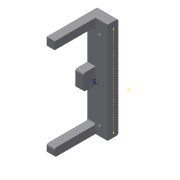
# Autodesk Inventor part: 30_Adapter_neje_to_cube_v3
Saved by Autodesk Inventor 2019.4 (Build 234330000, 330)
## iProperties
Created: 2021-04-09
Part Number: 30_Adapter_neje_to_cube_v3
Material: Generic
Document SubType Name: Modeling
Designer: UC2
Density: 1 g/cm^3
Appearance: Default
Author: UC2
Autodesk Inventor part; units mm, degrees
ref_plane "YZ Plane" through (0, 0, 0) normal (1, 0, 0) x (0, 1, 0)
ref_plane "XZ Plane" through (0, 0, 0) normal (0, 1, 0) x (-1, 0, 0)
sketch "Skizze1" plane through (0, 0, 0) normal (0, 0, 1) x (1, 0, 0)
  circle A0 centre (-23.32, -39.075) radius 2.355 construction
  circle A1 centre (-23.32, 39.075) radius 2.355 construction
  circle A2 centre (20.82, -6.975) radius 2 construction
  circle A3 centre (20.82, 7.075) radius 2 construction
  line L0 (32.82, 48.575) -> (-32.82, 48.575) construction
  arc A4 (-32.82, 48.575) -> (-34.82, 46.575) centre (-32.82, 46.575) ccw construction
  line L1 (-34.82, 46.575) -> (-34.82, -46.575) construction
  arc A5 (-34.82, -46.575) -> (-32.82, -48.575) centre (-32.82, -46.575) ccw construction
  line L2 (-32.82, -48.575) -> (32.82, -48.575) construction
  arc A6 (32.82, -48.575) -> (34.82, -46.575) centre (32.82, -46.575) ccw construction
  line L3 (34.82, -46.575) -> (34.82, 46.575) construction
  arc A7 (34.82, 46.575) -> (32.82, 48.575) centre (32.82, 46.575) ccw construction
  line L4 (-76.92, -46.575) -> (-35.32, -46.575) construction
  line L5 (-76.92, -40.695) -> (-76.92, -46.575) construction
  line L6 (-42.82, -40.695) -> (-76.92, -40.695) construction
  line L7 (-42.82, -0.875) -> (-42.82, -40.695) construction
  line L8 (-35.32, -0.875) -> (-42.82, -0.875) construction
  line L9 (-35.32, -46.575) -> (-35.32, -0.875) construction
  line L10 (-84.42, -46.575) -> (-76.92, -46.575) construction
  line L11 (-84.42, -0.875) -> (-84.42, -46.575) construction
  line L12 (-42.82, -0.875) -> (-84.42, -0.875) construction
  line L13 (-42.82, -6.755) -> (-42.82, -0.875) construction
  line L14 (-76.92, -6.755) -> (-42.82, -6.755) construction
  line L15 (-76.92, -46.575) -> (-76.92, -6.755) construction
  line L16 (-84.42, 3.425) -> (-76.92, 3.425) construction
  line L17 (-84.42, 49.125) -> (-84.42, 3.425) construction
  line L18 (-42.82, 49.125) -> (-84.42, 49.125) construction
  line L19 (-42.82, 43.245) -> (-42.82, 49.125) construction
  line L20 (-76.92, 43.245) -> (-42.82, 43.245) construction
  line L21 (-76.92, 3.425) -> (-76.92, 43.245) construction
  line L22 (-76.92, 3.425) -> (-35.32, 3.425) construction
  line L23 (-76.92, 9.305) -> (-76.92, 3.425) construction
  line L24 (-42.82, 9.305) -> (-76.92, 9.305) construction
  line L25 (-42.82, 49.125) -> (-42.82, 9.305) construction
  line L26 (-35.32, 49.125) -> (-42.82, 49.125) construction
  line L27 (-35.32, 3.425) -> (-35.32, 49.125) construction
  line L28 (-32.62, -40.5) -> (-32.62, -35.55) construction
  line L29 (-34.82, -40.5) -> (-32.62, -40.5) construction
  line L30 (-34.82, -35.55) -> (-32.62, -35.55) construction
  line L31 (-32.62, -11.9) -> (-32.62, -6.95) construction
  line L32 (-34.82, -11.9) -> (-32.62, -11.9) construction
  line L33 (-34.82, -6.95) -> (-32.62, -6.95) construction
  line L34 (-32.62, 9.5) -> (-32.62, 14.45) construction
  line L35 (-34.82, 9.5) -> (-32.62, 9.5) construction
  line L36 (-34.82, 14.45) -> (-32.62, 14.45) construction
  line L37 (-32.62, 38.1) -> (-32.62, 43.05) construction
  line L38 (-34.82, 38.1) -> (-32.62, 38.1) construction
  line L39 (-34.82, 43.05) -> (-32.62, 43.05) construction
  circle A8 centre (20.82, 7.075) radius 2 construction
  circle A9 centre (20.82, -6.975) radius 2 construction
  line L40 (13.32, -15) -> (17.82, -15) construction
  line L41 (13.32, -9.975) -> (13.32, -15) construction
  line L42 (17.32, -9.975) -> (13.32, -9.975) construction
  line L43 (17.32, -3.975) -> (17.32, -9.975) construction
  line L44 (13.32, -3.975) -> (17.32, -3.975) construction
  line L45 (13.32, 4.075) -> (13.32, -3.975) construction
  line L46 (17.32, 4.075) -> (13.32, 4.075) construction
  line L47 (17.32, 10.075) -> (17.32, 4.075) construction
  line L48 (13.32, 10.075) -> (17.32, 10.075) construction
  line L49 (13.32, 15) -> (13.32, 10.075) construction
  line L50 (17.82, 15) -> (13.32, 15) construction
  line L51 (17.82, 11) -> (17.82, 15) construction
  line L52 (23.82, 11) -> (17.82, 11) construction
  line L53 (23.82, 15) -> (23.82, 11) construction
  line L54 (28.32, 15) -> (23.82, 15) construction
  line L55 (28.32, 10.075) -> (28.32, 15) construction
  line L56 (24.32, 10.075) -> (28.32, 10.075) construction
  line L57 (24.32, 4.075) -> (24.32, 10.075) construction
  line L58 (28.32, 4.075) -> (24.32, 4.075) construction
  line L59 (28.32, -3.975) -> (28.32, 4.075) construction
  line L60 (24.32, -3.975) -> (28.32, -3.975) construction
  line L61 (24.32, -9.975) -> (24.32, -3.975) construction
  line L62 (28.32, -9.975) -> (24.32, -9.975) construction
  line L63 (28.32, -15) -> (28.32, -9.975) construction
  line L64 (23.82, -15) -> (28.32, -15) construction
  line L65 (23.82, -11) -> (23.82, -15) construction
  line L66 (17.82, -11) -> (23.82, -11) construction
  line L67 (17.82, -15) -> (17.82, -11) construction
  line L68 (-19.82, 48.575) -> (-34.82, 48.575)
  line L69 (-34.82, 48.575) -> (-34.82, -48.575)
  line L70 (-34.82, -48.575) -> (-19.82, -48.575)
  line L71 (-14.82, -43.575) -> (-14.82, 43.575)
  circle A10 centre (-23.32, 39.075) radius 2.455
  circle A11 centre (-23.32, -39.075) radius 2.255
  arc A12 (-19.82, -48.575) -> (-14.82, -43.575) centre (-19.82, -43.575) ccw
  arc A13 (-14.82, 43.575) -> (-19.82, 48.575) centre (-19.82, 43.575) ccw
  point P0 (0, 0)
  point P1 (-14.82, 48.575)
  point P2 (-14.82, -48.575)
  dimension "d1" = 0.1
  dimension "d2" = 0.1
  dimension "d8" = 20
  dimension "d9" = 5
  constraints: 24 end point, 9 horizontal, 5 point on line, 4 centre point, 4 point on circle, 4 tangent, 2 parallel, 1 collinear, 1 equal radius, 1 perpendicular, 1 vertical, 9 other
  measures "d1" radial gap between concentric circles of A1 A10
  measures "d2" radial gap between concentric circles of A0 A11
  measures "d8" distance between parallel lines of L71 L69
  measures "d9" radius of A12
extrude "Extrusion1" add sketch "Skizze1" along normal blind 5
sketch "Skizze2" plane through (0, 0, 5) normal (0, 0, 1) x (1, 0, 0)
  circle A0 centre (-23.32, 39.075) radius 2.455 construction
  circle A1 centre (-23.32, -39.075) radius 2.255 construction
  line L0 (-19.82, 48.575) -> (-34.82, 48.575) construction
  line L1 (-34.82, 48.575) -> (-34.82, -48.575) construction
  line L2 (-34.82, -48.575) -> (-19.82, -48.575) construction
  line L3 (-14.82, -43.575) -> (-14.82, 43.575) construction
  line L4 (-34.82, 48.575) -> (-29.82, 48.575)
  line L5 (-29.82, 48.575) -> (-29.82, -48.575)
  line L6 (-29.82, -48.575) -> (-34.82, -48.575)
  line L7 (-34.82, -48.575) -> (-34.82, 48.575)
  arc A2 (-19.82, -48.575) -> (-14.82, -43.575) centre (-19.82, -43.575) ccw projected
  arc A3 (-14.82, 43.575) -> (-19.82, 48.575) centre (-19.82, 43.575) ccw projected
  point P0 (0, 0)
  dimension "d5" = 5
  constraints: 8 end point, 2 parallel, 1 horizontal, 1 perpendicular, 1 point on line
  measures "d5" distance between parallel lines of L1 L5
ref_plane "Arbeitsebene1" through (-76.92, -46.575, 102.485) normal (0, 0, 1) x (1, 0, 0)
sketch "Sketch4" plane through (-34.82, -48.575, 0) normal (-1, 0, 0) x (0, 0, 1)
  line L0 (0, 0) -> (0, 97.15) projected
  line L1 (0, 0) -> (5, 0) projected
  line L2 (5, 97.15) -> (5, 0) construction
  line L3 (0, 97.15) -> (5, 97.15) projected
  circle A0 centre (41.935, 4.19) radius 2.475 projected
  circle A1 centre (13.335, 4.19) radius 2.475 projected
  circle A2 centre (13.335, 45.51) radius 2.475 projected
  circle A3 centre (13.335, 54.19) radius 2.475 projected
  circle A4 centre (13.335, 95.51) radius 2.475 projected
  circle A5 centre (41.935, 95.51) radius 2.475 projected
  line L4 (5, 0) -> (51, 0)
  line L5 (51, 0) -> (51, 8)
  line L6 (51, 8) -> (5, 8)
  line L7 (5, 8) -> (5, 0)
  line L8 (5, 8) -> (10.665, 8)
  line L9 (10.665, 8) -> (10.665, 99.5)
  line L10 (10.665, 99.5) -> (5, 99.5)
  line L11 (10.665, 99.5) -> (51, 99.5)
  line L12 (51, 99.5) -> (51, 91.82)
  line L13 (51, 91.82) -> (10.665, 91.82)
  line L14 (10.665, 91.82) -> (10.665, 99.5)
  line L15 (10.665, 41.82) -> (44.605, 41.82) projected
  line L16 (44.605, 57.88) -> (10.665, 57.88) projected
  line L17 (10.665, 41.82) -> (22.665, 41.82)
  line L18 (22.665, 41.82) -> (22.665, 57.88)
  line L19 (22.665, 57.88) -> (10.665, 57.88)
  line L20 (10.665, 57.88) -> (10.665, 41.82)
  line L21 (0, 0) -> (0, 97.15) projected
  line L22 (5, 99.5) -> (0, 99.5)
  line L23 (0, 99.5) -> (0, 0)
  line L24 (0, 0) -> (5, 0)
  line L25 (10.665, 91.82) -> (10.665, 57.88) construction
  line L26 (44.605, 91.82) -> (10.665, 91.82) construction
  line L27 (4.785, 99.7) -> (50.485, 99.7) construction
  line L28 (44.605, 91.82) -> (10.665, 91.82) construction
  circle A6 centre (6.975, 10.55) radius 2.475 projected
  circle A7 centre (6.975, 39.15) radius 2.475 projected
  circle A8 centre (6.975, 60.55) radius 2.475 projected
  circle A9 centre (6.975, 89.15) radius 2.475 projected
  line L29 (5, 97.15) -> (5, 0) projected
  line L30 (5, 40.6416) -> (5, 59.0584)
  line L31 (5, 59.0584) -> (5, 40.6416)
  line L32 (5, 62.0416) -> (5, 87.6584)
  line L33 (5, 90.6416) -> (5, 99.5)
  line L34 (5, 99.5) -> (5, 90.6416)
  line L35 (5, 87.6584) -> (5, 62.0416)
  line L36 (5, 37.6584) -> (5, 12.0416)
  line L37 (5, 9.0584) -> (5, 8)
  line L38 (5, 0) -> (5, 9.0584)
  line L39 (5, 12.0416) -> (5, 37.6584)
  point P0 (0, 48.575)
  dimension "d10" = 46
  dimension "d11" = 8
  dimension "d13" = 91.5
  dimension "d15" = 12
  constraints: 56 end point, 18 parallel, 8 point on circle, 5 horizontal, 5 perpendicular, 4 point on line, 2 coincident, 3 other
  measures "d10" distance of L6.end L5.end
  measures "d11" distance of L5.end L4.end
  measures "d13" distance of L9.end L8.end
  measures "d15" distance of L19.end L18.end
extrude "Extrusion3" add sketch "Sketch4" against normal up to surface (20 mm away) contours L0 L3 L29 A9 A8 A7 A6 L7 L1 | L23 L22 L33 L3 | L7 L6 L5 L4 | L33 L10 L9 L6 L29 A6 A7 A8 A9 | L29 A9 | L11 L12 L13 L9 | L9 L16 L18 L15 picked at (4.8333, 89.15)
fillet "Fillet1" radius 2 8 edges at (-24.82, 43.245, 10.665) (-24.82, 9.305, 22.665) (-24.82, -6.755, 22.665) (-24.82, -40.575, 10.665) (-24.82, -40.575, 51) (-24.82, -48.575, 51) (-24.82, 50.925, 0) (-24.82, -48.575, 0)
sketch "Sketch6" plane through (-34.82, -48.575, 2) normal (0, -1, 0) x (1, 0, 0)
  line L0 (20, 0) -> (0, 0) projected
  line L1 (20, 0) -> (20, 47) projected
  line L2 (0, 47) -> (20, 47) projected
  line L3 (0, 0) -> (0, 47) projected
  line L4 (20, 8.665) -> (0, 8.665) projected
  line L5 (0, 8.665) -> (20, 8.665) projected
  line L6 (21.8604, 55.0402) -> (8, 55.0402)
  line L7 (8, 55.0402) -> (8, 8.665)
  line L8 (8, 8.665) -> (21.8604, 8.665)
  line L9 (21.8604, 8.665) -> (21.8604, 55.0402)
  point P0 (34.82, -2)
  point P1 (12.8077, 8.665)
  dimension "d23" = 8
  constraints: 8 end point, 2 parallel, 1 horizontal, 1 perpendicular, 1 point on line
  measures "d23" distance between parallel lines of L7 L3
extrude "Extrusion5" cut sketch "Sketch6" against normal through all contours L4 L7 L2 L1 | L1 L2 L7 L6 L9 L8
sketch "Sketch7" plane through (-34.82, 43.245, 51) normal (-1, 0, 0) x (0, 0, 1)
  circle A0 centre (-37.665, -87.63) radius 2.475 projected
  circle A1 centre (-9.065, -87.63) radius 2.475 projected
  circle A2 centre (-37.665, -46.31) radius 2.475 projected
  circle A3 centre (-37.665, -37.63) radius 2.475 projected
  circle A4 centre (-37.665, 3.69) radius 2.475 projected
  point P0 (-51, -43.245)
sketch "Sketch8" plane through (-34.82, 43.245, 51) normal (-1, 0, 0) x (0, 0, 1)
  circle A0 centre (-44.025, -81.27) radius 2.475 projected
  circle A1 centre (-44.025, -52.67) radius 2.475 projected
  circle A2 centre (-44.025, -31.27) radius 2.475 projected
  circle A3 centre (-44.025, -2.67) radius 2.475 projected
  point P0 (-51, -43.245)
extrude "Extrusion6" cut sketch "Sketch8" against normal blind 6
chamfer "Chamfer1" distance 1 angle 45 18 edges at (-34.82, -44.385, 39.46) (-34.82, -44.385, 10.86) (-34.82, -3.065, 10.86) (-34.82, 5.615, 10.86) (-34.82, 46.935, 10.86) (-34.82, 46.935, 39.46) (-34.82, -9.425, 4.5) (-34.82, -11.7717, 7.7616) (-34.82, -7.0783, 7.7616) (-34.82, 11.975, 4.5) (-34.82, 9.6283, 7.7616) (-34.82, 14.3217, 7.7616) (-34.82, 38.2283, 7.7616) (-34.82, 42.9217, 7.7616) (-34.82, 40.575, 4.5) (-34.82, -38.025, 4.5) (-34.82, -40.3717, 7.7616) (-34.82, -35.6783, 7.7616)
sketch "Sketch9" plane through (-14.82, -48.575, 10.665) normal (1, 0, 0) x (0, 0, -1)
  line L0 (0, 0) -> (0, 99.5) projected
  line L1 (8.665, 0) -> (0, 0) projected
  arc A0 (8.665, 0) -> (10.665, 2) centre (8.665, 2) ccw projected
  line L2 (10.665, 97.5) -> (10.665, 2) projected
  arc A1 (10.665, 97.5) -> (8.665, 99.5) centre (8.665, 97.5) ccw projected
  line L3 (0, 99.5) -> (8.665, 99.5) projected
  arc A2 (5.665, 62.0416) -> (5.665, 59.0584) centre (3.69, 60.55) ccw projected
  line L4 (5.665, 59.0584) -> (5.665, 62.0416) projected
  arc A3 (5.665, 40.6416) -> (5.665, 37.6584) centre (3.69, 39.15) ccw projected
  line L5 (5.665, 37.6584) -> (5.665, 40.6416) projected
  line L6 (5.665, 87.6584) -> (5.665, 90.6416) projected
  arc A4 (5.665, 90.6416) -> (5.665, 87.6584) centre (3.69, 89.15) ccw projected
  arc A5 (5.665, 12.0416) -> (5.665, 9.0584) centre (3.69, 10.55) ccw projected
  line L7 (5.665, 9.0584) -> (5.665, 12.0416) projected
  point P0 (10.665, 48.575)
extrude "Extrusion7" add sketch "Sketch9" against normal up to surface (12 mm away) contours L4 A2 | L5 A3 | A4 L6 | L7 A5
sketch "Sketch10" plane through (0, 0, 0) normal (0, 0, -1) x (-1, 0, 0)
  circle A0 centre (23.32, -39.075) radius 2.355 construction
  circle A1 centre (23.32, 39.075) radius 2.355 construction
  circle A2 centre (-20.82, -6.975) radius 2 projected
  circle A3 centre (-20.82, 7.075) radius 2 projected
  line L0 (-32.82, 48.575) -> (32.82, 48.575) projected
  arc A4 (-32.82, 48.575) -> (-34.82, 46.575) centre (-32.82, 46.575) ccw projected
  line L1 (-34.82, -46.575) -> (-34.82, 46.575) projected
  arc A5 (-34.82, -46.575) -> (-32.82, -48.575) centre (-32.82, -46.575) ccw projected
  line L2 (32.82, -48.575) -> (-32.82, -48.575) projected
  arc A6 (32.82, -48.575) -> (34.82, -46.575) centre (32.82, -46.575) ccw projected
  line L3 (34.82, 46.575) -> (34.82, -46.575) projected
  arc A7 (34.82, 46.575) -> (32.82, 48.575) centre (32.82, 46.575) ccw projected
  circle A8 centre (16.82, -39.075) radius 1.4
  circle A9 centre (16.82, 39.075) radius 1.4
  line L4 (14.82, 48.925) -> (14.82, -46.575) projected
  point P0 (0, 0)
  dimension "d42" = 2.8
  dimension "d43" = 2.8
  dimension "d44" = 2
  dimension "d45" = 2
  constraints: 2 centre point
  measures "d42" diameter of A8
  measures "d43" diameter of A9
  measures "d44" distance from line of A8.centre L4
  measures "d45" distance from line of A9.centre L4
hole "Hole1" at (-23.32, -39.075, 0) at (-23.32, 39.075, 0) direction (0, 0, 1) diameter 2.8 end through all
sketch "Sketch11" plane through (-26.82, -48.575, 49) normal (1, 0, 0) x (0, 0, -1)
  circle A0 centre (7.065, 4.19) radius 2.475 projected
  circle A1 centre (35.665, 4.19) radius 2.475 projected
  arc A2 (-2, 2) -> (0, 0) centre (0, 2) ccw projected
  line L0 (38.335, 0) -> (0, 0) projected
  line L1 (38.335, 0) -> (38.335, 10) projected
  arc A3 (36.335, 8) -> (38.335, 10) centre (36.335, 10) ccw projected
  line L2 (0, 8) -> (36.335, 8) projected
  arc A4 (0, 8) -> (-2, 6) centre (0, 6) ccw projected
  line L3 (-2, 2) -> (-2, 6) projected
  line L4 (-2, 99.5) -> (38.335, 99.5) projected
  line L5 (-2, 91.82) -> (-2, 99.5) projected
  line L6 (36.335, 91.82) -> (-2, 91.82) projected
  arc A5 (38.335, 89.82) -> (36.335, 91.82) centre (36.335, 89.82) ccw projected
  line L7 (38.335, 89.82) -> (38.335, 99.5) projected
  circle A6 centre (7.065, 95.51) radius 2.475 projected
  circle A7 centre (35.665, 95.51) radius 2.475 projected
  line L8 (38.335, 41.82) -> (28.335, 41.82) projected
  line L9 (38.335, 41.82) -> (38.335, 57.88) projected
  line L10 (28.335, 57.88) -> (38.335, 57.88) projected
  arc A8 (28.335, 57.88) -> (26.335, 55.88) centre (28.335, 55.88) ccw projected
  line L11 (26.335, 43.82) -> (26.335, 55.88) projected
  arc A9 (26.335, 43.82) -> (28.335, 41.82) centre (28.335, 43.82) ccw projected
  circle A10 centre (35.665, 45.51) radius 2.475 projected
  circle A11 centre (35.665, 54.19) radius 2.475 projected
  point P0 (49, 48.575)
extrude "Extrusion8" add sketch "Sketch11" against normal blind 2 contours A0 | A1 | L3 A4 L2 A3 L1 L0 A2 | L4 L7 A5 L6 L5 | A6 | A7 | L8 A9 L11 A8 L10 L9 | A10 | A11
